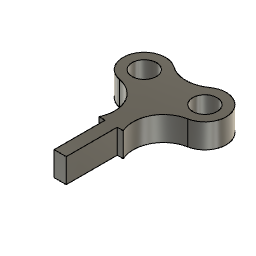
Model 13 (Autodesk Fusion 360 design; units mm, degrees)
Autodesk Fusion 360 part; units mm, degrees
sketch "Sketch1" plane through (0, 0, 0) normal (0, 0, 1) x (1, 0, 0)
  circle A0 centre (0, 0) radius 10
  line L0 (0, 0) -> (-50, 0) construction
  circle A1 centre (-50, 0) radius 10
  arc A2 (-39.7059, 14.1521) -> (-10.2941, 14.1521) centre (-25, 34.3693) ccw
  line L1 (9.4868, -28.4605) -> (9.4868, -40.9605)
  line L2 (-50, 0) -> (-50, 17.5) construction
  line L3 (-50, 17.5) -> (0, 17.5) construction
  line L4 (-25, 17.5) -> (-25, -94.314) construction
  line L5 (-25, -94.314) -> (-20, -94.314)
  line L6 (-25, -94.314) -> (-30, -94.314)
  line L7 (-20, -94.314) -> (-20, -52.314)
  line L8 (-30, -94.314) -> (-30, -52.314)
  line L9 (-20, -52.314) -> (-15, -52.314)
  line L10 (-30, -52.314) -> (-35, -52.314)
  arc A3 (-35, -52.314) -> (-53.163, -17.2118) centre (-57.6816, -41.8) ccw
  arc A4 (3.163, -17.2118) -> (-15, -52.314) centre (7.6816, -41.8) ccw
  arc A5 (-39.7059, 14.1521) -> (-53.163, -17.2118) centre (-50, 0) ccw
  arc A6 (3.163, -17.2118) -> (-10.2941, 14.1521) centre (0, 0) ccw
  dimension "d6" = 20
  dimension "d7" = 35
  dimension "d8" = 50
  dimension "d9" = 20
  dimension "d10" = 35
  dimension "d11" = 50
  dimension "d14" = 111.814
  dimension "d15" = 5
  dimension "d16" = 5
  dimension "d17" = 42
  dimension "d18" = 42
  dimension "d19" = 5
  dimension "d20" = 5
  dimension "d22" = 50
  dimension "d23" = 50
  constraint coincident A0.centre L0.start
  constraint horizontal L0
  constraint coincident L0.end A1.centre
  constraint concentric A1 A5
  constraint tangent A2 A6
  constraint tangent A2 A5
  constraint vertical L1
  constraint coincident L2.end A5
  constraint perpendicular L0 L2
  constraint coincident L3.end A6
  constraint tangent L3 A6
  constraint midpoint L3 L4.start
  constraint perpendicular L0 L4
  constraint perpendicular L4 L5
  constraint perpendicular L4 L6
  constraint perpendicular L5 L7
  constraint perpendicular L6 L8
  constraint perpendicular L7 L9
  constraint perpendicular L8 L10
  constraint tangent A3 A5
  constraint tangent A4 A6
  measures "d6" diameter of A0
  measures "d7" diameter of A6
  measures "d8" distance of A0.centre L0.end
  measures "d9" diameter of A1
  measures "d10" diameter of A5
  measures "d11" diameter of A2
  measures "d14" distance of L4.start L4.end
  measures "d15" distance of L4.end L5.end
  measures "d16" distance of L4.end L6.end
  measures "d17" distance of L5.end L7.end
  measures "d18" distance of L6.end L8.end
  measures "d19" distance of L7.end L9.end
  measures "d20" distance of L8.end L10.end
  measures "d22" diameter of A3
  measures "d23" diameter of A4
extrude "Extrude1" add sketch "Sketch1" along normal blind 20
